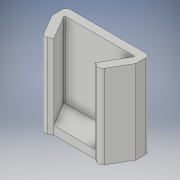
# Autodesk Inventor part: rail
Saved by Autodesk Inventor 2019 (Build 230136000, 136)
## iProperties
Created: 2019-02-07
Part Number: rail
Material: Generic
Document SubType Name: Modeling
Designer: jmc
Density: 1 g/cm^3
Appearance: Default
Author: jmc
Autodesk Inventor part; units mm, degrees
ref_plane "YZ Plane" through (0, 0, 0) normal (1, 0, 0) x (0, 1, 0)
ref_plane "XZ Plane" through (0, 0, 0) normal (0, 1, 0) x (-1, 0, 0)
ref_plane "XY Plane" through (0, 0, 0) normal (0, 0, 1) x (1, 0, 0)
sketch "Sketch1" plane through (0, 0, 0) normal (0, 0, 1) x (1, 0, 0)
  line L0 (5, -10) -> (-5, -10)
  line L1 (-5, -10) -> (-5, 10)
  line L2 (-5, 10) -> (5, 10)
  line L3 (5, 10) -> (5, -10)
  line L4 (5, -10) -> (-5, 10) construction
  line L5 (-5, -10) -> (5, 10) construction
  point P0 (0, 0)
  dimension "d0" = 10
  dimension "d1" = 20
  constraints: 12 end point, 2 midpoint, 2 parallel, 1 horizontal, 1 perpendicular
  measures "d0" distance of L1.end L2.end
  measures "d1" distance of L0.end L1.end
extrude "Extrusion1" add sketch "Sketch1" along normal blind 2
sketch "Sketch2" plane through (0, 0, 0) normal (0, 0, -1) x (-1, 0, 0)
  line L0 (-5, -10) -> (5, -10) construction
  line L1 (5, -10) -> (5, 10) construction
  line L2 (5, 10) -> (-5, 10) construction
  line L3 (-5, 10) -> (-5, -10) construction
  line L4 (-5, -10) -> (-5, 10) projected
  line L5 (-5, 10) -> (-10, 10)
  line L6 (-10, 10) -> (-10, -10)
  line L7 (-10, -10) -> (-5, -10)
  line L8 (-5, -10) -> (-5, 10)
  line L9 (5, 10) -> (5, -10) projected
  line L10 (5, 10) -> (10, 10)
  line L11 (10, 10) -> (10, -10)
  line L12 (10, -10) -> (5, -10)
  line L13 (5, -10) -> (5, 10)
  line L14 (5, -10) -> (-5, -10) projected
  point P0 (0, 0)
  dimension "d4" = 5
  dimension "d5" = 5
  constraints: 16 end point, 4 parallel, 2 horizontal, 2 perpendicular, 1 collinear, 1 point on line
  measures "d4" distance of L7.end L6.end
  measures "d5" distance of L11.end L12.end
extrude "Extrusion2" add sketch "Sketch2" against normal blind 10
sketch "Sketch3" plane through (-10, 10, 0) normal (0, 1, 0) x (1, 0, 0)
  line L0 (0, 0) -> (20, 0) construction
  line L1 (0, 0) -> (0, -10) construction
  line L2 (5, -10) -> (0, -10) construction
  line L3 (5, -2) -> (5, -10) construction
  line L4 (15, -2) -> (5, -2) construction
  line L5 (15, -2) -> (15, -10) construction
  line L6 (20, -10) -> (15, -10) construction
  line L7 (20, 0) -> (20, -10) construction
  line L8 (5, -8) -> (1.6755, -2.3008)
  line L9 (1.8482, -2) -> (5, -2)
  line L10 (15, -8) -> (18.3245, -2.3008)
  line L11 (18.1518, -2) -> (15, -2)
  arc A0 (1.8482, -2) -> (1.6755, -2.3008) centre (1.8482, -2.2) ccw
  arc A1 (18.3245, -2.3008) -> (18.1518, -2) centre (18.1518, -2.2) ccw
  line L12 (5, -2) -> (5, -10) projected
  line L13 (5, -8) -> (5, -2)
  line L14 (15, -2) -> (15, -8)
  line L15 (15, -2) -> (15, -10) projected
  point P0 (10, 0)
  point P1 (1.5, -2)
  point P2 (18.5, -2)
  dimension "d9" = 2
  dimension "d10" = 3.5
  dimension "d11" = 3.5
  dimension "d12" = 2
  dimension "d13" = 0.2
  constraints: 12 end point, 6 point on line, 4 point on circle, 4 tangent, 2 centre point, 2 collinear, 1 equal radius, 1 horizontal
  measures "d9" distance of L8.start L2.start
  measures "d10" distance of point (1.5, -2) L3.start
  measures "d11" distance of point (18.5, -2) L4.start
  measures "d12" distance of L10.start L5.end
  measures "d13" radius of A0
extrude "Extrusion3" cut sketch "Sketch3" against normal through all
sketch "Sketch4" plane through (-10, 10, 0) normal (0, 1, 0) x (1, 0, 0)
  line L0 (0, -3.3978) -> (3.2724, -9.0077)
  line L1 (5, -10) -> (0, -10) projected
  line L2 (5, -8) -> (1.6755, -2.3008) projected
  line L3 (1.8482, -2) -> (18.1518, -2) projected
  line L4 (0, 0) -> (20, 0) projected
  line L5 (0, 0) -> (0, -10) projected
  line L6 (0, -3.3978) -> (0, -10)
  line L7 (20, -3.3381) -> (16.7016, -8.9926)
  line L8 (20, -10) -> (15, -10) projected
  line L9 (18.3245, -2.3008) -> (15, -8) projected
  line L10 (20, 0) -> (20, -10) projected
  line L11 (20, -3.3381) -> (20, -10)
  line L12 (5, -8) -> (3.2724, -9.0077)
  line L13 (15, -8) -> (15, -10) projected
  line L14 (15, -8) -> (16.7016, -8.9926)
  line L15 (5, -8) -> (5, -10) projected
  line L16 (5, -8) -> (5, -10)
  point P0 (10, 0)
  dimension "d16" = 2
  dimension "d17" = 2
  constraints: 14 end point, 2 collinear, 2 parallel, 2 perpendicular, 2 point on line, 1 vertical
  measures "d16" distance between parallel lines of L0 L2
  measures "d17" distance between parallel lines of L3 L4
extrude "Extrusion4" cut sketch "Sketch4" against normal through all
sketch "Sketch6" plane through (-10, -10, 0) normal (0, -1, 0) x (1, 0, 0)
  line L0 (1.6755, 2.3008) -> (5, 8) projected
  line L1 (18.1518, 2) -> (1.8482, 2) projected
  line L2 (15, 8) -> (18.3245, 2.3008) projected
  arc A0 (18.1518, 2) -> (18.3245, 2.3008) centre (18.1518, 2.2) ccw projected
  arc A1 (1.6755, 2.3008) -> (1.8482, 2) centre (1.8482, 2.2) ccw projected
  line L3 (3.2724, 9.0077) -> (5, 8) projected
  line L4 (5, 8) -> (15, 8)
  point P0 (10, 0)
  constraints: 2 end point, 1 horizontal
extrude "Extrusion6" add sketch "Sketch6" against normal blind 2
fillet "Fillet1" [suppressed]
fillet "Fillet2" radius 1 4 edges at (6.7016, 0, 8.9926) (-10, 0, 0) (10, 0, 0) (-6.7276, 0, 9.0077)
equation "\"d11\" = d10"
equation "\"d12\" = d9"
body "Solid1"
